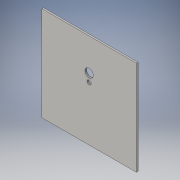
# Autodesk Inventor part: ClawPlate
Saved by Autodesk Inventor 2016 (Build 200138000, 138)
## iProperties
Created: 2016-01-25
Part Number: ClawPlate
Material: Generic
Document SubType Name: Modeling
Designer: Mentor1102
Density: 1 g/cm^3
Appearance: Default
Author: Mentor1102
Autodesk Inventor part; units mm, degrees
ref_plane "YZ Plane" through (0, 0, 0) normal (1, 0, 0) x (0, 1, 0)
ref_plane "XZ Plane" through (0, 0, 0) normal (0, 1, 0) x (-1, 0, 0)
ref_plane "XY Plane" through (0, 0, 0) normal (0, 0, 1) x (1, 0, 0)
sketch "Sketch1" plane through (0, 0, 0) normal (0, 0, 1) x (1, 0, 0)
  line L0 (0, 0) -> (177.8, 0)
  line L1 (177.8, 0) -> (177.8, 177.8)
  line L2 (177.8, 177.8) -> (0, 177.8)
  line L3 (0, 177.8) -> (0, 0)
  dimension "d0" = 177.8
  dimension "d1" = 177.8
  constraints: 8 end point, 2 parallel, 1 horizontal, 1 perpendicular
  measures "d0" distance of L2.end L1.end
  measures "d1" distance of L1.end L0.end
extrude "Extrusion1" add sketch "Sketch1" along normal blind 3.175
sketch "Sketch2" plane through (0, 0, 3.175) normal (0, 0, 1) x (1, 0, 0)
  line L0 (0, 0) -> (177.8, 0) projected
  line L1 (177.8, 0) -> (177.8, 177.8) projected
  line L2 (177.8, 177.8) -> (0, 177.8) construction
  line L3 (0, 177.8) -> (0, 0) projected
  line L4 (177.8, 177.8) -> (0, 177.8) construction
  line L5 (88.9, 177.8) -> (76.2, 177.8) construction
  line L6 (88.9, 177.8) -> (101.6, 177.8) construction
  line L7 (76.2, 177.8) -> (76.2, 127) construction
  line L8 (76.2, 127) -> (101.6, 127) construction
  line L9 (101.6, 177.8) -> (101.6, 127) construction
  line L10 (88.9, 127) -> (88.9, 107.95) construction
  circle A0 centre (88.9, 117.475) radius 9.525 construction
  circle A1 centre (88.9, 117.475) radius 7.874
  dimension "d4" = 12.7
  dimension "d5" = 12.7
  dimension "d6" = 50.8
  dimension "d7" = 19.05
  dimension "d8" = 15.748
  constraints: 12 end point, 3 midpoint, 3 vertical, 2 point on line, 1 centre point, 1 coincident, 1 perpendicular, 1 vertical alignment, 2 other
  measures "d4" distance of L5.start L5.end
  measures "d5" distance of L5.start L6.end
  measures "d6" distance of L5.end L7.end
  measures "d7" distance of L10.start L10.end
  measures "d8" diameter of A1
extrude "Extrusion2" cut sketch "Sketch2" against normal through all
sketch "Sketch3" plane through (0, 0, 3.175) normal (0, 0, 1) x (1, 0, 0)
  circle A0 centre (88.9, 117.475) radius 7.874 projected
  line L0 (0, 0) -> (177.8, 0) projected
  line L1 (177.8, 0) -> (177.8, 177.8) projected
  line L2 (177.8, 177.8) -> (0, 177.8) projected
  line L3 (0, 177.8) -> (0, 0) projected
  circle A1 centre (88.9, 117.475) radius 10.16 construction
  line L4 (88.9, 117.475) -> (88.9, 107.315) construction
  line L5 (88.9, 107.315) -> (88.9, 102.235) construction
  circle A2 centre (88.9, 102.235) radius 3.9116
  dimension "d11" = 20.32
  dimension "d12" = 5.08
  dimension "d13" = 7.8232
  constraints: 4 end point, 2 coincident, 2 vertical, 1 centre point, 1 vertical alignment, 2 other
  measures "d12" distance of L4.end L5.end
  measures "d13" diameter of A2
extrude "Extrusion3" cut sketch "Sketch3" against normal through all contours A2
body "Solid1"
